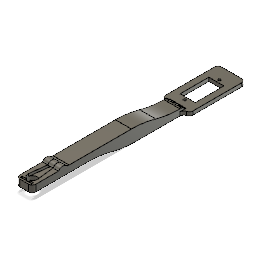
SOAR_Arm_Long-v1 (Autodesk Fusion 360 design; units mm, degrees)
Autodesk Fusion 360 part; units mm, degrees
note: some values were not read from the file. Chosen so that the rebuilt part matches the saved one: which face or edge a step refers to; which pieces of a blend or face edit are solid.
sketch "Sketch1" plane through (0, 0, 0) normal (0, 1, 0) x (1, 0, 0)
  line L0 (0, 0) -> (13, 0)
  line L1 (13, 0) -> (13, -26)
  line L2 (13, -26) -> (0, -26)
  line L3 (0, -26) -> (0, 0)
  line L4 (2, -23) -> (11, -23)
  line L5 (11, -23) -> (11, -4)
  line L6 (11, -4) -> (2, -4)
  line L7 (2, -4) -> (2, -23)
  line L8 (6.5, -23) -> (6.5, -19.2)
  circle A0 centre (6.5, -19.2) radius 3.8
  circle A1 centre (6.5, -4) radius 2
  line L9 (4.5, -4) -> (2.7272, -18.7464)
  line L10 (8.5, -4) -> (10.2728, -18.7464)
  line L11 (0, 0) -> (13, 0)
  line L12 (13, 0) -> (13, 5.1268)
  line L13 (13, 5.1268) -> (0, 5.1268)
  line L14 (0, 5.1268) -> (0, 0)
  line L15 (5, -23.5) -> (8, -23.5)
  line L16 (8, -23.5) -> (8, -22.5)
  line L17 (8, -22.5) -> (5, -22.5)
  line L18 (5, -22.5) -> (5, -23.5)
  line L19 (2, -23) -> (11, -23)
  line L20 (11, -23) -> (11, -24.5)
  line L21 (11, -24.5) -> (2, -24.5)
  line L22 (2, -24.5) -> (2, -23)
  dimension "d1" = 13
  dimension "d2" = 26
  dimension "d3" = 3.8
  dimension "d4" = 4
  constraint horizontal L0
  constraint vertical L1
  constraint horizontal L2
  constraint vertical L3
  constraint coincident L0.start L3.end
  constraint horizontal L4
  constraint vertical L5
  constraint horizontal L6
  constraint vertical L7
  constraint midpoint L4 L8.start
  constraint perpendicular L4 L8
  constraint coincident L8.end A0.centre
  constraint coincident L8.start A0
  constraint midpoint L6 A1.centre
  constraint coincident L6 L9.start
  constraint coincident A1 L9.start
  constraint coincident A0 L9.end
  constraint tangent A0 L9
  constraint coincident A1 L10.start
  constraint coincident L6 L10.start
  constraint coincident A0 L10.end
  constraint tangent A0 L10
  constraint horizontal L11
  constraint vertical L12
  constraint horizontal L13
  constraint vertical L14
  constraint horizontal L15
  constraint vertical L16
  constraint horizontal L17
  constraint vertical L18
  constraint horizontal L19
  constraint vertical L20
  constraint horizontal L21
  constraint vertical L22
  measures "d1" distance of L0.start L0.end
  measures "d2" distance of L0.start L2.end
  measures "d3" distance of L8.start L8.end
  measures "d4" diameter of A1
extrude "Extrude13" add sketch "Sketch1" along normal blind 5.5 contours L0 L1 L2 L3 L11 | L4 L6 L7 A0 L9 L18 L19 | L4 L5 L6 A0 L10 L16 L19 makes body 1
extrude "Extrude14" add sketch "Sketch1" along normal blind 3.5 contours L6 A1 | L6 A1 | A0 A1 L9 L10 bodies 1
sketch "Sketch7" plane through (0, 5.5, 0) normal (0, 1, 0) x (-1, 0, 0)
  line L0 (-8, 22.6914) -> (-8, 23)
  line L1 (-8, 23) -> (-11, 23)
  line L2 (-11, 23) -> (-11, 24.5)
  line L3 (-11, 24.5) -> (-2, 24.5)
  line L4 (-2, 24.5) -> (-2, 23)
  line L5 (-2, 23) -> (-5, 23)
  line L6 (-5, 23) -> (-5, 22.6914)
  arc A0 (-2.7272, 18.7464) -> (-5, 22.6914) centre (-6.5, 19.2) ccw
  line L7 (-2.7272, 18.7464) -> (-4.5, 4)
  arc A1 (-8.5, 4) -> (-4.5, 4) centre (-6.5, 4) ccw
  line L8 (-8.5, 4) -> (-10.2728, 18.7464)
  arc A2 (-8, 22.6914) -> (-10.2728, 18.7464) centre (-6.5, 19.2) ccw
  line L9 (0, 0) -> (0, 26)
  line L10 (0, 26) -> (-13, 26)
  line L11 (-13, 26) -> (-13, 0)
  line L12 (-13, 0) -> (0, 0)
  line L13 (0, 0) -> (-13, 0)
  line L14 (-13, 0) -> (-13, 5)
  line L15 (-13, 5) -> (0, 5)
  line L16 (0, 5) -> (0, 0)
  dimension "d49" = 13
  dimension "d50" = 5
  constraint horizontal L13
  constraint vertical L14
  constraint horizontal L15
  constraint vertical L16
  constraint coincident L9.start L12.end
  measures "d49" distance of L9.start L11.end
  measures "d50" distance of L9.start L15.end
extrude "Extrude15" add sketch "Sketch7" along normal blind 2 contours L7 A1 L8 L15 | L7 A1 L8 L9 L11 L12 L13 L14 L15 L16 bodies 1
sketch "Sketch8" plane through (0, 0, 0) normal (0, 1, 0) x (1, 0, 0)
  line L0 (0, 0) -> (13, 0)
  line L1 (13, 0) -> (13, 100)
  line L2 (13, 100) -> (0, 100)
  line L3 (0, 100) -> (0, 0)
  dimension "d53" = 100
  constraint horizontal L0
  constraint vertical L1
  constraint horizontal L2
  constraint vertical L3
  constraint coincident L0.start L3.end
  measures "d53" distance of L0.start L2.end
extrude "Extrude16" add sketch "Sketch8" along normal blind 5.5 bodies 1
sketch "Sketch9" plane through (0, 0, 0) normal (0, 1, 0) x (1, 0, 0)
  line L0 (0, 100) -> (12.5884, 100)
  line L1 (12.5884, 100) -> (12.5884, 90)
  line L2 (12.5884, 90) -> (0, 90)
  line L3 (0, 90) -> (0, 100)
  dimension "d56" = 10
  constraint horizontal L0
  constraint vertical L1
  constraint horizontal L2
  constraint vertical L3
  measures "d56" distance of L0.start L2.end
sketch "Sketch10" plane through (0, -5, 0) normal (0, -1, 0) x (1, 0, 0)
  line L0 (0, -90) -> (0, -100)
  line L1 (0, -100) -> (12.5884, -100)
  line L2 (12.5884, -100) -> (12.5884, -90)
  line L3 (0.5884, -100) -> (0.5884, -132.5)
  line L4 (0.5884, -132.5) -> (12.5884, -132.5)
  line L5 (12.5884, -132.5) -> (12.5884, -100)
  line L6 (17.5884, -140) -> (17.5884, -95)
  line L7 (17.5884, -95) -> (-4.4116, -95)
  line L8 (-4.4116, -95) -> (-4.4116, -140)
  line L9 (-4.4116, -140) -> (17.5884, -140)
  line L10 (12.5884, -100) -> (0.5884, -100)
  line L11 (12.5884, -100) -> (0.5884, -100)
  line L12 (0.5884, -100) -> (0.5884, -104.8)
  line L13 (0.5884, -104.8) -> (12.5884, -104.8)
  line L14 (12.5884, -104.8) -> (12.5884, -100)
  line L15 (12.5884, -132.5) -> (0.5884, -132.5)
  line L16 (0.5884, -132.5) -> (0.5884, -127.7)
  line L17 (0.5884, -127.7) -> (12.5884, -127.7)
  line L18 (12.5884, -127.7) -> (12.5884, -132.5)
  line L19 (6.5884, -100) -> (6.5884, -132.5)
  line L20 (6.5884, -100) -> (6.5884, -104.8)
  circle A0 centre (6.5884, -102.4) radius 1
  line L21 (6.5884, -127.7) -> (6.5884, -132.5)
  circle A1 centre (6.5884, -130.1) radius 1
  dimension "d60" = 12
  dimension "d61" = 32.5
  dimension "d63" = 12
  dimension "d64" = 4.8
  dimension "d65" = 12
  dimension "d66" = 4.8
  dimension "d67" = 2
  dimension "d68" = 2
  constraint vertical L3
  constraint horizontal L4
  constraint vertical L5
  constraint coincident L1.end L2.start
  constraint parallel L5 L6
  constraint parallel L3 L8
  constraint parallel L4 L9
  constraint perpendicular L0 L10
  constraint horizontal L11
  constraint vertical L12
  constraint horizontal L13
  constraint vertical L14
  constraint horizontal L15
  constraint vertical L16
  constraint horizontal L17
  constraint vertical L18
  constraint midpoint L10 L19.start
  constraint midpoint L4 L19.end
  constraint midpoint L13 L20.end
  constraint midpoint L20 A0.centre
  constraint midpoint L17 L21.start
  constraint midpoint L21 A1.centre
  measures "d60" distance of L1.end L3.start
  measures "d61" distance of L1.end L4.end
  measures "d63" distance of L1.end L3.start
  measures "d64" distance of L1.end L13.end
  measures "d65" distance of L4.end L3.end
  measures "d66" distance of L4.end L17.end
  measures "d67" diameter of A0
  measures "d68" diameter of A1
extrude "Extrude18" add sketch "Sketch10" against normal blind 3 separate body contours L0 L1 L2 L7 L10 L11 | L0 L1 L2 L3 L4 L5 L6 L7 L8 L9 L12 L14 L15 L16 L18 | L1 L3 L10 L11 L12 L13 L19 L20 A0 | L1 L5 L10 L11 L13 L14 L19 L20 A0 | L3 L4 L15 L16 L17 L19 L21 A1 | L4 L5 L15 L17 L18 L19 L21 A1 makes body 2
extrude "Extrude19" cut 1 faces at (8.6667, 1.8333, -100) along direction (0, 0, 1) blind 5 on bodies 1 bodies 1
sketch "Sketch11" plane through (0, 0, 0) normal (0, -1, 0) x (1, 0, 0)
  line L0 (0, -95) -> (13, -95)
  line L1 (13, -95) -> (13, 26)
  line L2 (13, 26) -> (0, 26)
  line L3 (0, 26) -> (0, -95)
  line L4 (8, 23) -> (8, 22.6914)
  arc A0 (5, 22.6914) -> (8, 22.6914) centre (6.5, 19.2) ccw
  line L5 (5, 22.6914) -> (5, 23)
  line L6 (5, 23) -> (2, 23)
  line L7 (2, 23) -> (2, 24.5)
  line L8 (2, 24.5) -> (11, 24.5)
  line L9 (11, 24.5) -> (11, 23)
  line L10 (11, 23) -> (8, 23)
  line L11 (13, -95) -> (0, -95)
  line L12 (0, -95) -> (0, -65)
  line L13 (0, -65) -> (13, -65)
  line L14 (13, -65) -> (13, -95)
  line L15 (0, -65) -> (13, -65)
  line L16 (13, -65) -> (13, -45)
  line L17 (13, -45) -> (0, -45)
  line L18 (0, -45) -> (0, -65)
  dimension "d73" = 20
  constraint horizontal L11
  constraint vertical L12
  constraint horizontal L13
  constraint vertical L14
  constraint coincident L3 L12.end
  constraint coincident L0.end L1.start
  constraint horizontal L15
  constraint vertical L16
  constraint horizontal L17
  constraint vertical L18
  measures "d73" distance of L12.end L17.end
extrude "Extrude20" add sketch "Sketch11" along normal blind 5 contours L0 L1 L3 L11 L12 L13 L14 L15 | L1 L3 L13 L15 L16 L17 L18 bodies 1 2
extrude "Extrude21" cut sketch "Sketch11" against normal blind 9 contours L0 L1 L3 L11 L12 L13 L14 L15 bodies 1
fillet "Fillet11" radius 70 4 edges at (6.5, 0, -65) (6.5, 5.5, -65) (6.5, 0, -45) (6.5, -5, -45) on bodies 1
fillet "Fillet12" radius 3 8 edges at (17.5884, -3.5, -95) (13, -3.5, -95) (17.5884, -3.5, -140) (-4.4116, -3.5, -140) (-4.4116, -3.5, -95) (0, -3.5, -95) (0, 2.75, 26) (13, 2.75, 26) on bodies 1
fillet "Fillet13" radius 2 2 edges at (6.5, 0, -95) (6.5, -2, -95) on bodies 1
fillet "Fillet14" radius 4 3 edges at (6.5, 7.5, 0) (6.5, 7.5, 5) (6.5, 5.5, 0) on bodies 1
